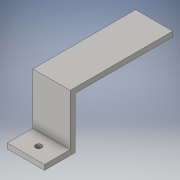
# Autodesk Inventor part: Battery Mount
Saved by Autodesk Inventor 2016 (Build 200138000, 138)
## iProperties
Created: 2017-10-13
Part Number: Battery Mount
Material: Generic
Document SubType Name: Modeling
Designer: Student
Density: 1 g/cm^3
Appearance: Default
Author: Student
Autodesk Inventor part; units mm, degrees
ref_plane "YZ Plane" through (0, 0, 0) normal (1, 0, 0) x (0, 1, 0)
ref_plane "XZ Plane" through (0, 0, 0) normal (0, 1, 0) x (-1, 0, 0)
ref_plane "XY Plane" through (0, 0, 0) normal (0, 0, 1) x (1, 0, 0)
sketch "Sketch1" plane through (0, 0, 0) normal (1, 0, 0) x (0, 1, 0)
  line L0 (0.979, 1.6933) -> (0.979, 14.3933)
  line L1 (0.979, 14.3933) -> (3.519, 14.3933)
  line L2 (3.519, 14.3933) -> (3.519, 1.6933)
  line L3 (3.519, 1.6933) -> (25.3145, 1.6933)
  line L4 (26.379, -0.8467) -> (0.979, -0.8467)
  line L5 (0.979, -0.8467) -> (0.979, 1.6933)
  line L6 (25.3145, 1.6933) -> (26.379, 1.6933)
  line L7 (26.379, 1.6933) -> (28.919, 1.6933)
  line L8 (28.919, 1.6933) -> (28.919, -49.1067)
  line L9 (28.919, -49.1067) -> (26.379, -49.1067)
  line L10 (26.379, -49.1067) -> (26.379, -0.8467)
  point P0 (0, 0)
  dimension "d0" = 12.7
  dimension "d1" = 12.7
  dimension "d2" = 2.54
  dimension "d11" = 25.4
  dimension "d12" = 2.54
  dimension "d13" = 50.8
  constraints: 22 end point, 3 horizontal, 2 parallel, 2 perpendicular, 2 vertical, 1 point on line
  measures "d0" distance of L2.end L1.end
  measures "d1" distance of L0.start L0.end
  measures "d2" distance of L0.end L1.end
  measures "d11" distance of L4.start L4.end
  measures "d12" distance of L6.end L7.end
  measures "d13" distance of L7.end L8.end
extrude "Extrusion1" add sketch "Sketch1" along normal blind 18.415
sketch "Sketch2" plane through (0, 3.519, 14.3933) normal (0, 1, 0) x (1, 0, 0)
  circle A0 centre (9.2075, 6.35) radius 1.5
  line L0 (18.415, 12.7) -> (18.415, 0) projected
  line L1 (0, 0) -> (18.415, 0) projected
  point P0 (0, 14.3933)
  point P1 (18.415, 6.35)
  point P2 (9.2075, 0)
  dimension "d8" = 3
  constraints: 2 midpoint, 1 centre point, 1 horizontal alignment, 1 vertical alignment
  measures "d8" diameter of A0
extrude "Extrusion2" cut sketch "Sketch2" against normal blind 18.415
body "Solid1"
